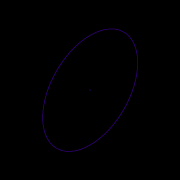
# Autodesk Inventor part: pipe
Saved by Autodesk Inventor 2019 (Build 230136000, 136)
## iProperties
Created: 2019-01-06
Part Number: pipe
Material: Generic
Document SubType Name: Modeling
Designer: MJ
Density: 1 g/cm^3
Appearance: Default
Author: MJ
Autodesk Inventor part; units mm, degrees
ref_plane "YZ Plane" through (0, 0, 0) normal (1, 0, 0) x (0, 1, 0)
ref_plane "XZ Plane" through (0, 0, 0) normal (0, 1, 0) x (-1, 0, 0)
ref_plane "XY Plane" through (0, 0, 0) normal (0, 0, 1) x (1, 0, 0)
sketch "Sketch1" plane through (0, 0, 0) normal (1, 0, 0) x (0, 1, 0)
  circle A0 centre (0, 10) radius 5
  line L0 (0, -9.7682) -> (0, 29.6525)
  point P0 (0, 0)
  dimension "d1" = 10
  dimension "d2" = 10
  constraints: 2 end point, 2 point on line, 1 centre point, 1 vertical
  measures "d1" diameter of A0
  measures "d2" distance of point (0, 0) A0.centre
extrude "Extrusion1" add sketch "Sketch1" along normal mid plane 10
body "Solid1"
